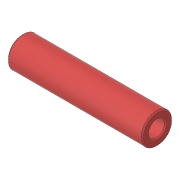
# Autodesk Inventor part: AR-2622
Saved by Autodesk Inventor 2019.4 (Build 234330000, 330)
## iProperties
Created: 2019-11-17
Part Number: AR-2622
Material: 一般
Document SubType Name: Modeling
Designer: y6tada
Density: 1 g/cm^3
Appearance: 滑らか - 赤
Author: y6tada
Autodesk Inventor part; units mm, degrees
ref_plane "YZ Plane" through (0, 0, 0) normal (1, 0, 0) x (0, 1, 0)
ref_plane "XZ Plane" through (0, 0, 0) normal (0, 1, 0) x (-1, 0, 0)
ref_plane "XY Plane" through (0, 0, 0) normal (0, 0, 1) x (1, 0, 0)
sketch "スケッチ1" plane through (0, 0, 0) normal (1, 0, 0) x (0, 1, 0)
  circle A0 centre (0, 0) radius 2.5
  circle A1 centre (0, 0) radius 1.3
  dimension "d0" = 5
  dimension "d1" = 2.6
  constraints: 2 centre point, 2 coincident
  measures "d0" diameter of A0
  measures "d1" diameter of A1
extrude "押し出し1" add sketch "スケッチ1" along normal mid plane 22
chamfer "面取り1" distance 0.2 angle 45 4 edges at (11, -1.3, 0) (11, -2.5, 0) (-11, -1.3, 0) (-11, -2.5, 0)
